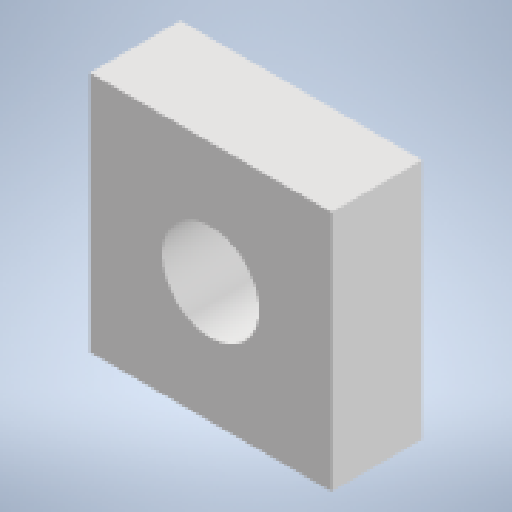
# Autodesk Inventor part: Soporte gomas
Saved by Autodesk Inventor 2024 (Build 280153000, 153)
## iProperties
Created: 2025-03-01
Part Number: Soporte gomas
Material: Genérico
Document SubType Name: Modeling
Designer: sergi
Density: 1 g/cm^3
Appearance: Valor por defecto
Author: sergi
Autodesk Inventor part; units mm, degrees
ref_plane "YZ Plane" through (0, 0, 0) normal (1, 0, 0) x (0, 1, 0)
ref_plane "XZ Plane" through (0, 0, 0) normal (0, 1, 0) x (-1, 0, 0)
ref_plane "XY Plane" through (0, 0, 0) normal (0, 0, 1) x (1, 0, 0)
sketch "Boceto1" plane through (0, 0, 0) normal (0, 0, 1) x (1, 0, 0)
  circle A0 centre (0, 37) radius 2.1 projected
  circle A1 centre (0, -37) radius 2.1 projected
  line L0 (4, 41) -> (4, -41) projected
  line L1 (-4, 41) -> (4, 41) projected
  line L2 (-4, -41) -> (-4, 41) projected
  line L3 (4, -41) -> (-4, -41) projected
  line L4 (4, 41) -> (-4, 41)
  line L5 (-4, 41) -> (-4, 33)
  line L6 (-4, 33) -> (4, 33)
  line L7 (4, 33) -> (4, 41)
  circle A2 centre (0, 37) radius 1.6
  point P0 (0, 0)
  dimension "d2" = 3.2
  constraints: 8 end point, 2 parallel, 1 centre point, 1 coincident, 1 horizontal, 1 perpendicular, 1 point on line
  measures "d2" diameter of A2
ref_plane "Plano de trabajo1" through (-9.1, 23, 5.1) normal (0, 0, 1) x (1, 0, 0)
extrude "Extrusión1" add sketch "Boceto1" along normal blind 3 contours A0 | L0 L6 L2 L1
